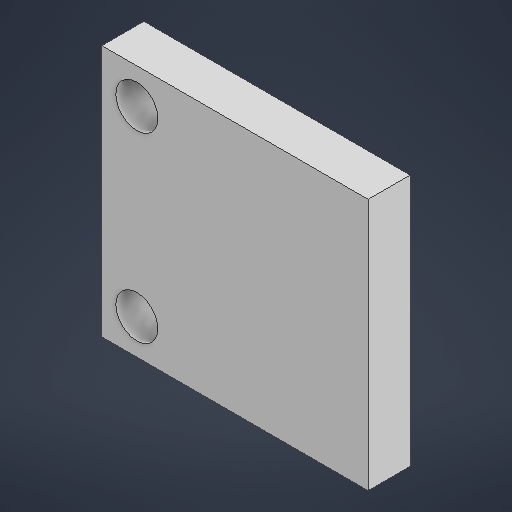
# Autodesk Inventor part: TOF - VL6180X Fermion SEN0427
Saved by Autodesk Inventor 2026.2 (Build 302298010, 298A)
## iProperties
Created: 2026-03-17
Part Number: TOF - VL6180X Fermion SEN0427
Material: Générique
Document SubType Name: Modeling
Designer: cleml
Density: 1 g/cm^3
Appearance: Par défaut
Author: cleml
Autodesk Inventor part; units mm, degrees
ref_plane "YZ Plane" through (0, 0, 0) normal (1, 0, 0) x (0, 1, 0)
ref_plane "XZ Plane" through (0, 0, 0) normal (0, 1, 0) x (-1, 0, 0)
ref_plane "XY Plane" through (0, 0, 0) normal (0, 0, 1) x (1, 0, 0)
sketch "Esquisse1" plane through (0, 0, 0) normal (0, 0, 1) x (1, 0, 0)
  line L0 (0, 0) -> (19, 0)
  line L1 (19, 0) -> (19, 18)
  line L2 (19, 18) -> (0, 18)
  line L3 (0, 18) -> (0, 0)
  dimension "d0" = 19
  dimension "d1" = 18
  constraints: 8 end point, 2 parallel, 1 horizontal, 1 perpendicular
  measures "d0" distance of L1.end L2.end
  measures "d1" distance of L0.end L1.end
extrude "Extrusion1" add sketch "Esquisse1" along normal blind 3
sketch "Esquisse2" plane through (0, 0, 3) normal (0, 0, 1) x (1, 0, 0)
  line L0 (19, 18) -> (0, 18) projected
  line L1 (0, 18) -> (0, 0) projected
  circle A0 centre (2.5, 2.5) radius 1.5
  circle A1 centre (2.5, 15.5) radius 1.5
  dimension "d4" = 13
  dimension "d5" = 2.5
  dimension "d6" = 2.5
  dimension "d7" = 2.5
  dimension "d8" = 3
  dimension "d9" = 3
  constraints: 2 centre point, 2 coincident
  measures "d4" distance of point (2.5, 15.5) point (2.5, 2.5)
  measures "d5" distance from line of L0 point (2.5, 15.5)
  measures "d6" distance from line of L1 point (2.5, 2.5)
  measures "d7" distance from line of L1 point (2.5, 15.5)
  measures "d8" diameter of A0
  measures "d9" diameter of A1
extrude "Extrusion2" cut sketch "Esquisse2" against normal through all
equation "\"d7\" = d6"
